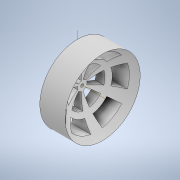
# Autodesk Inventor part: 2022plateForBall
Saved by Autodesk Inventor 2022.2 (Build 262287000, 287)
## iProperties
Created: 2020-01-14
Part Number: 2022plateForBall
Material: Generic
Document SubType Name: Modeling
Designer: steele
Density: 1 g/cm^3
Appearance: Default
Author: steele
Autodesk Inventor part; units mm, degrees
ref_plane "YZ Plane" through (0, 0, 0) normal (1, 0, 0) x (0, 1, 0)
ref_plane "XZ Plane" through (0, 0, 0) normal (0, 1, 0) x (-1, 0, 0)
ref_plane "XY Plane" through (0, 0, 0) normal (0, 0, 1) x (1, 0, 0)
sketch "Sketch4" plane through (0, 0, 0) normal (0, 0, 1) x (1, 0, 0)
  line L0 (0, 0) -> (101.6, 0) construction
  arc A0 (68.2819, 101.6) -> (12.7, 0) centre (133.35, 0) ccw
  line L1 (12.7, 0) -> (12.7, 96.7762) construction
  line L2 (0, 0) -> (0, 101.6)
  line L3 (0, 101.6) -> (68.2819, 101.6)
  line L4 (0, 0) -> (12.7, 0)
  dimension "d11" = 101.6
  dimension "d12" = 12.7
  dimension "d13" = 101.6
  dimension "d14" = 241.3
  constraints: 10 end point, 2 point on circle, 2 point on line, 2 vertical, 1 centre point, 1 collinear, 1 horizontal, 1 perpendicular, 1 tangent
  measures "d11" distance of L0.start L0.end
  measures "d12" distance from line of L0.start L1
  measures "d13" distance of L0.start L2.end
  measures "d14" diameter of A0
revolve "Revolution2" add sketch "Sketch4" angle 360 about axis through (0, 0, 0) along (1, 0, 0)
sketch "Sketch6" plane through (0, 0, 0) normal (-1, 0, 0) x (0, 0, 1)
  point P0 (0, 0)
  point P1 (0, 0)
  constraints: 1 coincident
hole "Hole1" at (0, 0, 0) direction (1, 0, 0) diameter 7.9248 end through all
sketch "Sketch10" plane through (0, 0, 0) normal (-1, 0, 0) x (0, 0, 1)
  circle A0 centre (0, 0) radius 101.6 projected
  circle A1 centre (0, 0) radius 3.9624 construction
  line L0 (0, 0) -> (-101.6, 0) construction
  circle A2 centre (0, 0) radius 101.6 projected
  circle A3 centre (0, 0) radius 12.7
  arc A4 (-83.5387, 30.4056) -> (-83.5387, -30.4056) centre (0, 0) ccw
  arc A5 (-59.6705, 21.7183) -> (-59.6705, -21.7183) centre (0, 0) ccw
  arc A6 (-47.7364, 17.3746) -> (-47.7364, -17.3746) centre (0, 0) ccw
  line L1 (-11.9341, 4.3437) -> (-47.7364, 17.3746)
  line L2 (-59.6705, 21.7183) -> (-83.5387, 30.4056)
  line L3 (-11.9341, -4.3437) -> (-47.7364, -17.3746)
  line L4 (-59.6705, -21.7183) -> (-83.5387, -30.4056)
  dimension "d58" = 25.4
  dimension "d59" = 12.7
  dimension "d60" = 12.7
  dimension "d61" = 38.1
  constraints: 10 end point, 8 point on circle, 4 centre point, 4 coincident, 2 horizontal alignment, 1 horizontal, 1 other
  measures "d58" diameter of A3
  measures "d60" radial gap between concentric circles of A6 A5
  measures "d61" radial gap between concentric circles of A6 A3
extrude "Extrusion7" cut sketch "Sketch10" against normal through all contours A3 L3 A6 L1 | L2 A5 L4 A4
pattern_circular "Circular Pattern4" count 6 over 360 about axis through (-10, 0, 0) along (1, 0, 0) of "Extrusion7"
body "Solid3"
